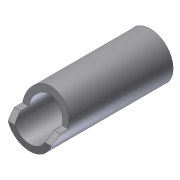
# Autodesk Inventor part: MPS Mouse Tube
Saved by Autodesk Inventor 2012 SP2 (Build 160219200, 219)
## iProperties
Created: 2014-07-09
Material: Default
Vendor: HHMI: JFRC - ID&F
Document SubType Name: Modeling
Designer: arnoldj
Density: 1 g/cm^3
RuleStatus: InUse
AfterDocSave0: file://Part Number Cleaner
DESIGN DEPARTMENT: HHMI: JFRC - ID&F
ALTERED ITEM PART NUMBER: N/A
ALTERED ITEM VENDOR: N/A
ALTERED ITEM DESCRIPTION: N/A
Revision Number: 0
Autodesk Inventor part; units mm, degrees
ref_plane "YZ Plane" through (0, 0, 0) normal (1, 0, 0) x (0, 1, 0)
ref_plane "XZ Plane" through (0, 0, 0) normal (0, 1, 0) x (-1, 0, 0)
ref_plane "XY Plane" through (0, 0, 0) normal (0, 0, 1) x (1, 0, 0)
sketch "Sketch1" plane through (0, 0, 0) normal (0, 0, 1) x (1, 0, 0)
  circle A0 centre (0, 0) radius 13.97
  circle A1 centre (0, 0) radius 19.05
  dimension "d0" = 27.94
  dimension "d1" = 38.1
  constraints: 2 centre point, 2 coincident
  measures "d0" diameter of A0
  measures "d1" diameter of A1
extrude "Extrusion1" add sketch "Sketch1" along normal blind 100.33
sketch "Sketch2" plane through (0, 0, 0) normal (1, 0, 0) x (0, 1, 0)
  line L0 (-19.05, 100.33) -> (19.05, 100.33) projected
  line L1 (19.05, 0) -> (19.05, 100.33) projected
  line L2 (-0.0364, 100.33) -> (-0.0364, 87.2336)
  line L3 (-0.0364, 87.2336) -> (19.05, 82.7907)
  line L4 (-0.0364, 100.33) -> (19.05, 100.33)
  point P0 (0, 0)
  constraints: 6 end point, 2 point on line, 1 collinear, 1 parallel
extrude "Extrusion2" cut sketch "Sketch2" along normal through all both and the other way through all
chamfer "Chamfer1" distance 6.35 angle 45 2 edges at (16.51, -0.0364, 100.33) (-16.51, -0.0364, 100.33)
body "Solid1"
